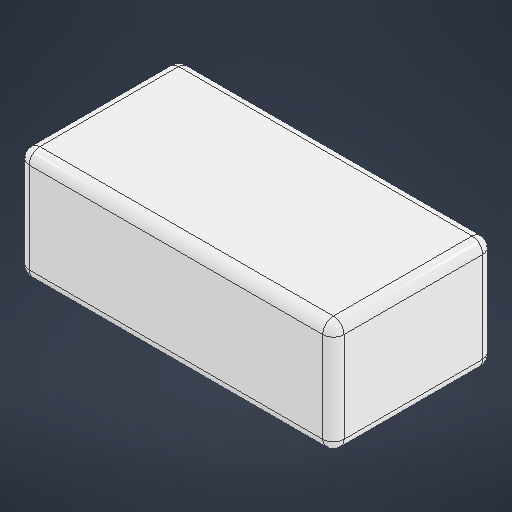
# Autodesk Inventor part: 12V Akku
Saved by Autodesk Inventor 2025.2 (Build 292293000, 293)
## iProperties
Created: 2025-03-28
Part Number: 12V Akku
Material: Generisch
Document SubType Name: Modeling
Designer: Faabs
Density: 1 g/cm^3
Appearance: Weiß
Author: Faabs
Autodesk Inventor part; units mm, degrees
ref_plane "YZ Plane" through (0, 0, 0) normal (1, 0, 0) x (0, 1, 0)
ref_plane "XZ Plane" through (0, 0, 0) normal (0, 1, 0) x (-1, 0, 0)
ref_plane "XY Plane" through (0, 0, 0) normal (0, 0, 1) x (1, 0, 0)
sketch "Skizze1" plane through (0, 0, 0) normal (0, 0, 1) x (1, 0, 0)
  line L0 (-29.5, -15) -> (29.5, -15)
  line L1 (29.5, -15) -> (29.5, 15)
  line L2 (29.5, 15) -> (-29.5, 15)
  line L3 (-29.5, 15) -> (-29.5, -15)
  line L4 (-29.5, -15) -> (29.5, 15) construction
  line L5 (29.5, -15) -> (-29.5, 15) construction
  point P0 (0, 0)
  dimension "d0" = 59
  dimension "d1" = 30
  constraints: 12 end point, 2 midpoint, 2 parallel, 1 horizontal, 1 perpendicular
  measures "d0" distance of L1.end L2.end
  measures "d1" distance of L0.end L1.end
extrude "Extrusion1" add sketch "Skizze1" along normal mid plane 21
fillet "Rundung1" radius 2 12 edges at (29.5, 0, -10.5) (29.5, -15, 0) (0, -15, -10.5) (0, 15, -10.5) (29.5, 15, 0) (29.5, 0, 10.5) (-29.5, 0, -10.5) (-29.5, -15, 0) (-29.5, 0, 10.5) (-29.5, 15, 0) (0, -15, 10.5) (0, 15, 10.5)
